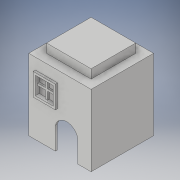
# Autodesk Inventor part: House Model
Saved by Autodesk Inventor 2018 (Build 220112000, 112)
## iProperties
Created: 2018-12-03
Part Number: House Model
Material: Generic
Document SubType Name: Modeling
Designer: Administrator
Density: 1 g/cm^3
Appearance: Default
Author: Administrator
Autodesk Inventor part; units mm, degrees
ref_plane "YZ Plane" through (0, 0, 0) normal (1, 0, 0) x (0, 1, 0)
ref_plane "XZ Plane" through (0, 0, 0) normal (0, 1, 0) x (-1, 0, 0)
ref_plane "XY Plane" through (0, 0, 0) normal (0, 0, 1) x (1, 0, 0)
sketch "Sketch1" plane through (0, 0, 0) normal (0, 0, 1) x (1, 0, 0)
  line L0 (0, 0) -> (177.8, 0)
  line L1 (177.8, 0) -> (177.8, 203.2)
  line L2 (177.8, 203.2) -> (0, 203.2)
  line L3 (0, 203.2) -> (0, 0)
  line L4 (0, 203.2) -> (25.4, 203.2) construction
  line L5 (177.8, 203.2) -> (203.2, 203.2) construction
  line L6 (0, 203.2) -> (177.8, 203.2)
  line L7 (177.8, 203.2) -> (177.8, 228.6)
  line L8 (177.8, 228.6) -> (0, 228.6)
  line L9 (0, 228.6) -> (0, 203.2)
  dimension "d0" = 177.8
  dimension "d1" = 203.2
  dimension "d6" = 177.8
  dimension "d7" = 25.4
  constraints: 20 end point, 4 horizontal, 4 parallel, 2 perpendicular
  measures "d0" distance of L2.end L1.end
  measures "d1" distance of L1.end L0.end
  measures "d6" distance of L8.end L7.end
  measures "d7" distance of L7.end L6.end
extrude "Extrusion1" add sketch "Sketch1" along normal blind 177.8
sketch "Sketch2" plane through (0, 0, 177.8) normal (0, 0, 1) x (1, 0, 0)
  line L0 (177.8, 228.6) -> (0, 228.6) projected
  line L1 (0, 228.6) -> (177.8, 228.6)
  line L2 (177.8, 228.6) -> (177.8, 203.2)
  line L3 (177.8, 203.2) -> (0, 203.2)
  line L4 (0, 203.2) -> (0, 228.6)
  point P0 (0, 0)
  dimension "d10" = 177.8
  dimension "d11" = 25.4
  constraints: 8 end point, 2 parallel, 1 horizontal, 1 perpendicular
  measures "d10" distance of L2.end L3.end
  measures "d11" distance of L1.end L2.end
extrude "Extrusion2" cut sketch "Sketch2" against normal blind 25.4
sketch "Sketch3" plane through (177.8, 0, 0) normal (1, 0, 0) x (0, 0, -1)
  line L0 (0, 0) -> (0, 228.6) projected
  line L1 (-177.8, 0) -> (-177.8, 203.2) projected
  line L2 (0, 228.6) -> (-177.8, 228.6)
  line L3 (-177.8, 228.6) -> (-177.8, 203.2)
  line L4 (-177.8, 203.2) -> (0, 203.2)
  line L5 (0, 203.2) -> (0, 228.6)
  dimension "d14" = 177.8
  dimension "d15" = 25.4
  constraints: 8 end point, 2 parallel, 1 horizontal, 1 perpendicular
  measures "d14" distance of L4.end L1.end
  measures "d15" distance of L1.end L2.end
extrude "Extrusion3" cut sketch "Sketch3" against normal blind 25.4
sketch "Sketch4" plane through (0, 0, 0) normal (0, 0, -1) x (-1, 0, 0)
  line L0 (0, 228.6) -> (0, 0) projected
  line L1 (-152.4, 203.2) -> (-177.8, 203.2) projected
  line L2 (0, 228.6) -> (-177.8, 228.6)
  line L3 (-177.8, 228.6) -> (-177.8, 203.2)
  line L4 (-177.8, 203.2) -> (0, 203.2)
  line L5 (0, 203.2) -> (0, 228.6)
  dimension "d18" = 177.8
  dimension "d19" = 25.4
  constraints: 8 end point, 2 parallel, 1 horizontal, 1 perpendicular
  measures "d18" distance of L4.end L1.end
  measures "d19" distance of L1.end L2.end
extrude "Extrusion4" cut sketch "Sketch4" against normal blind 25.4
sketch "Sketch5" plane through (0, 0, 0) normal (-1, 0, 0) x (0, 0, 1)
  line L0 (177.8, 228.6) -> (0, 228.6)
  line L1 (0, 228.6) -> (0, 203.2)
  line L2 (0, 203.2) -> (177.8, 203.2)
  line L3 (177.8, 203.2) -> (177.8, 228.6)
  line L4 (177.8, 203.2) -> (177.8, 0) projected
  line L5 (25.4, 228.6) -> (152.4, 228.6) projected
  point P0 (0, 0)
  dimension "d22" = 177.8
  dimension "d23" = 25.4
  dimension "d24" = 0
  dimension "d25" = 0
  constraints: 8 end point, 2 parallel, 1 horizontal, 1 perpendicular
  measures "d22" distance of L2.end L1.end
  measures "d23" distance of L1.end L0.end
  measures "d24" distance between parallel lines of L4 L3
  measures "d25" distance between parallel lines of L5 L0
extrude "Extrusion5" cut sketch "Sketch5" against normal blind 25.4
shell "Shell1" thickness 5.08 removed faces 1 at (59.2667, 0, 59.2667)
sketch "Sketch6" plane through (0, 0, 177.8) normal (0, 0, 1) x (1, 0, 0)
  line L0 (25.4, 165.1) -> (76.2, 165.1)
  line L1 (76.2, 165.1) -> (76.2, 114.3)
  line L2 (76.2, 114.3) -> (25.4, 114.3)
  line L3 (25.4, 114.3) -> (25.4, 165.1)
  line L4 (177.8, 203.2) -> (0, 203.2) projected
  line L5 (0, 203.2) -> (0, 0) projected
  line L6 (47.625, 165.1) -> (53.975, 165.1)
  line L7 (53.975, 114.3) -> (47.625, 114.3)
  line L8 (76.2, 142.875) -> (76.2, 136.525)
  line L9 (25.4, 136.525) -> (25.4, 142.875)
  line L10 (47.625, 114.3) -> (47.625, 136.525)
  line L11 (47.625, 142.875) -> (47.625, 165.1)
  line L12 (25.4, 142.875) -> (47.625, 142.875)
  line L13 (53.975, 142.875) -> (76.2, 142.875)
  line L14 (53.975, 165.1) -> (53.975, 142.875)
  line L15 (53.975, 136.525) -> (53.975, 114.3)
  line L16 (76.2, 136.525) -> (53.975, 136.525)
  line L17 (47.625, 136.525) -> (25.4, 136.525)
  line L18 (82.55, 171.45) -> (19.05, 171.45)
  line L19 (19.05, 171.45) -> (19.05, 107.95)
  line L20 (19.05, 107.95) -> (82.55, 107.95)
  line L21 (82.55, 107.95) -> (82.55, 171.45)
  dimension "d29" = 50.8
  dimension "d30" = 50.8
  dimension "d31" = 38.1
  dimension "d32" = 25.4
  dimension "d33" = 6.35
  dimension "d34" = 50.8
  dimension "d36" = 50.8
  dimension "d37" = 6.35
  dimension "d39" = 6.35
  constraints: 40 end point, 14 parallel, 6 perpendicular, 4 horizontal, 2 point on line, 3 other
  measures "d29" distance of L1.end L2.end
  measures "d30" distance of L0.end L1.end
  measures "d31" distance between parallel lines of L4 L0
  measures "d32" distance between parallel lines of L5 L3
  measures "d33" distance of L7.start L7.end
  measures "d34" distance of L6.end L7.start
  measures "d36" distance of L8.end L9.start
  measures "d37" distance of L8.start L8.end
  measures "d39" distance between parallel lines of L0 L18
extrude "Extrusion6" cut sketch "Sketch6" against normal blind 25.4 contours L0 L11 L12 L3 | L0 L1 L13 L14 | L17 L10 L2 L3 | L1 L2 L15 L16
extrude "Extrusion7" add sketch "Sketch6" along normal blind 6.35
sketch "Sketch7" plane through (0, 0, 177.8) normal (0, 0, 1) x (1, 0, 0)
  line L0 (0, 0) -> (177.8, 0) projected
  line L1 (76.2, 0) -> (139.7, 0)
  line L2 (139.7, 0) -> (139.7, 88.9)
  line L3 (139.7, 88.9) -> (76.2, 88.9)
  line L4 (76.2, 88.9) -> (76.2, 0)
  line L5 (177.8, 0) -> (177.8, 203.2) projected
  line L6 (76.2, 0) -> (76.2, 63.5)
  arc A0 (139.7, 63.5) -> (76.2, 63.5) centre (107.95, 56.3852) ccw
  dimension "d44" = 63.5
  dimension "d45" = 88.9
  dimension "d46" = 38.1
  dimension "d47" = 63.5
  dimension "d48" = 32.5374
  constraints: 10 end point, 3 point on line, 2 parallel, 2 point on circle, 1 centre point, 1 horizontal, 1 perpendicular
  measures "d44" distance of L3.end L2.end
  measures "d45" distance of L2.end L1.end
  measures "d46" distance between parallel lines of L5 L2
  measures "d47" distance of L1.start L6.end
  measures "d48" radius of A0
extrude "Extrusion8" cut sketch "Sketch7" against normal blind 6.35 contours L4 A0 L3 L2 L0 | A0 L3
body "Solid1"
